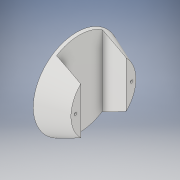
# Autodesk Inventor part: 1st base
Saved by Autodesk Inventor 2017 (Build 210142000, 142)
## iProperties
Created: 2020-02-20
Part Number: 1st base
Material: UHMW, White
Document SubType Name: Modeling
Designer: S346852600
Density: 0.94 g/cm^3
Appearance: Smooth - White
Author: S346852600
Autodesk Inventor part; units mm, degrees
ref_plane "YZ Plane" through (0, 0, 0) normal (1, 0, 0) x (0, 1, 0)
ref_plane "XZ Plane" through (0, 0, 0) normal (0, 1, 0) x (-1, 0, 0)
ref_plane "XY Plane" through (0, 0, 0) normal (0, 0, 1) x (1, 0, 0)
sketch "Sketch1" plane through (0, 0, 0) normal (1, 0, 0) x (0, 1, 0)
  circle A0 centre (0.7746, 0) radius 41.021
  point P0 (0, 0)
  dimension "d1" = 82.042
  constraints: 1 centre point
  measures "d1" diameter of A0
extrude "Extrusion1" add sketch "Sketch1" along normal blind 25.4 draft -22
sketch "Sketch3" plane through (25.4, 0.7746, 0) normal (1, 0, 0) x (0, 0, -1)
  circle A0 centre (0, 0) radius 30.7587 projected
  line L0 (0, 0) -> (-21.4773, 0)
  line L1 (-21.4773, 0) -> (-21.4773, 41.021)
  line L2 (-21.4773, 41.021) -> (0, 41.021)
  line L3 (0, 41.021) -> (0, 0)
  line L4 (30.7587, 0) -> (21.6147, 0)
  line L5 (-21.4773, 41.021) -> (21.6147, 41.021)
  line L6 (21.6147, 41.021) -> (21.6147, -46.8819)
  line L7 (21.6147, -46.8819) -> (-21.4773, -46.8819)
  line L8 (-21.4773, -46.8819) -> (-21.4773, 41.021)
  point P0 (0, -0.7746)
  dimension "d5" = 9.144
  constraints: 18 end point, 4 parallel, 3 horizontal, 2 perpendicular, 1 horizontal alignment, 1 other
  measures "d5" distance of L4.start L4.end
extrude "Extrusion2" cut sketch "Sketch3" against normal blind 22.86 contours L6 A0 L8 L0 L3 | A0 L3 L5 L6 | L6 L7 L8 A0 | L3 L0 L1 A0 | A0 L1 L2 L3
sketch "Sketch5" plane through (0, 0.7746, 0) normal (-1, 0, 0) x (0, 0, 1)
  circle A0 centre (0, -0.7746) radius 6.35
  dimension "d13" = 12.7
  constraints: 1 centre point, 1 coincident
  measures "d13" diameter of A0
extrude "Extrusion4" cut sketch "Sketch5" against normal blind 1.27
sketch "Sketch6" plane through (25.4, 0, 0) normal (1, 0, 0) x (0, 0, -1)
  circle A0 centre (-26.5573, 0.7715) radius 1.27
  circle A1 centre (-26.5573, 0.7715) radius 1.27
  point P0 (0, 0)
  constraints: 2 centre point, 1 coincident, 1 concentric
extrude "Extrusion5" cut sketch "Sketch6" against normal blind 1.27
sketch "Sketch8" plane through (25.4, 0, 0) normal (1, 0, 0) x (0, 0, -1)
  circle A0 centre (26.6947, 0.7715) radius 1.27 projected
  point P0 (0, 0)
extrude "Extrusion7" cut sketch "Sketch8" against normal blind 1.27
body "Solid1"
